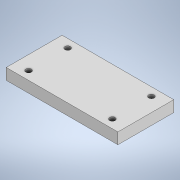
# Autodesk Inventor part: bracket
Saved by Autodesk Inventor 2021 (Build 250183000, 183)
## iProperties
Created: 2020-12-19
Part Number: bracket
Material: Generic
Document SubType Name: Modeling
Designer: awitc
Density: 1 g/cm^3
Appearance: Default
Author: awitc
Autodesk Inventor part; units mm, degrees
ref_plane "YZ Plane" through (0, 0, 0) normal (1, 0, 0) x (0, 1, 0)
ref_plane "XZ Plane" through (0, 0, 0) normal (0, 1, 0) x (-1, 0, 0)
ref_plane "XY Plane" through (0, 0, 0) normal (0, 0, 1) x (1, 0, 0)
sketch "Sketch1" plane through (0, 0, 0) normal (0, 1, 0) x (-1, 0, 0)
  line L0 (20, 10) -> (0, 10)
  line L1 (0, 10) -> (20, 10)
  line L2 (20, 10) -> (20, 0)
  line L3 (20, 0) -> (0, 0)
  line L4 (0, 0) -> (0, 10)
  line L5 (0, 10) -> (2.5, 10)
  circle A0 centre (2.5, 8.5) radius 0.5
  circle A1 centre (2.5, 1.5) radius 0.5
  circle A2 centre (17.5, 1.5) radius 0.5
  circle A3 centre (17.5, 8.5) radius 0.5
  point P0 (0, 0)
  point P1 (10, 0)
  point P2 (10, 0)
  point P3 (16.8377, 0)
  point P4 (20, 10)
  dimension "d0" = 20
  dimension "d1" = 2.5
  dimension "d2" = 1
  dimension "d3" = 1
  dimension "d4" = 1
  dimension "d5" = 1
  constraints: 12 end point, 4 centre point, 2 parallel, 1 horizontal, 1 perpendicular, 1 point on line
  measures "d0" distance of L2.end L3.end
  measures "d1" distance of L0.end L5.end
  measures "d2" diameter of A0
  measures "d3" diameter of A1
  measures "d4" diameter of A2
  measures "d5" diameter of A3
extrude "Extrusion1" add sketch "Sketch1" along normal blind 2
body "Solid1"
